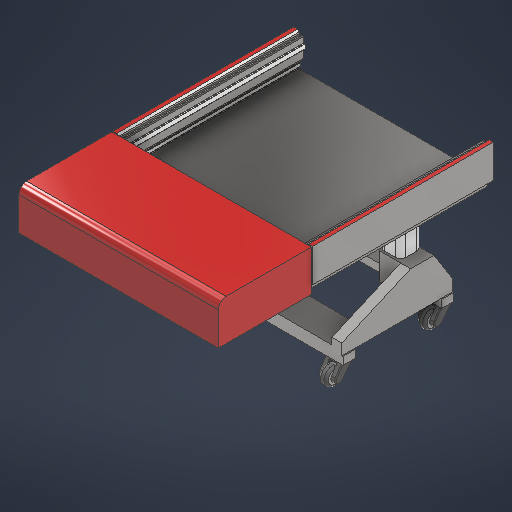
# Autodesk Inventor part: SACMI PH1500 POWER FEED SYSTEM
Saved by Autodesk Inventor 2025 (Build 290162000, 162)
## iProperties
Created: 2024-05-03
Part Number: SACMI PH1500 POWER FEED SYSTEM
Material: Generic
Document SubType Name: Modeling
Designer: zulet
Density: 1 g/cm^3
Appearance: Steel - Polished
Author: zulet
Autodesk Inventor part; units mm, degrees
ref_plane "YZ Plane" through (0, 0, 0) normal (1, 0, 0) x (0, 1, 0)
ref_plane "XZ Plane" through (0, 0, 0) normal (0, 1, 0) x (-1, 0, 0)
ref_plane "XY Plane" through (0, 0, 0) normal (0, 0, 1) x (1, 0, 0)
sketch "Sketch1" plane through (0, 0, 0) normal (0, 1, 0) x (-1, 0, 0)
  line L0 (700, -390) -> (-700, -390)
  line L1 (-700, -390) -> (-700, -500)
  line L2 (-700, -500) -> (700, -500)
  line L3 (700, -500) -> (700, -390)
  line L4 (0, 0) -> (0, -500) construction
  line L5 (0, 0) -> (-700, 0) construction
  line L6 (700, 390) -> (-700, 390)
  line L7 (-700, 390) -> (-700, 500)
  line L8 (-700, 500) -> (700, 500)
  line L9 (700, 500) -> (700, 390)
  point P0 (0, 500)
  dimension "d0" = 1400
  dimension "d1" = 500
  dimension "d2" = 110
  constraints: 20 end point, 5 symmetric about line, 2 horizontal, 2 parallel, 1 midpoint, 1 perpendicular, 1 point on line, 1 vertical
  measures "d0" distance of L1.end L2.end
  measures "d1" distance of L4.start L4.end
  measures "d2" distance between parallel lines of L0 L2
extrude "Extrusion1" add sketch "Sketch1" along normal blind 70
sketch "Sketch2" plane through (700, 0, 500) normal (1, 0, 0) x (0, 0, -1)
  line L0 (-1602.6406, 1986.5614) -> (1424.7743, 1986.5614) construction
  line L1 (1424.7743, 1986.5614) -> (1424.7743, -298.4008) construction
  line L2 (1424.7743, -298.4008) -> (-1602.6406, -298.4008) construction
  line L3 (-1602.6406, -298.4008) -> (-1602.6406, 1986.5614) construction
  line L4 (1917.7715, 602.0909) -> (1917.7715, -167.9091) construction
  line L5 (890, 70) -> (1000, 70) projected
  line L6 (0, 0) -> (0, 70) projected
  line L7 (1000, 70) -> (0, 70)
  line L8 (0, 70) -> (0, 170)
  line L9 (0, 170) -> (620, 440)
  line L10 (620, 440) -> (830, 440)
  line L11 (830, 440) -> (1000, 170)
  line L12 (1000, 170) -> (1000, 70)
  point P0 (500, 0)
  dimension "d10" = 770
  dimension "d30" = 2284.9623
  dimension "d45" = 100
  dimension "d46" = 210
  dimension "d47" = 270
  dimension "d48" = 620
  dimension "d49" = 100
  constraints: 14 end point, 2 parallel, 2 perpendicular, 1 horizontal, 1 vertical, 2 other
  measures "d10" distance of L4.start L4.end
  measures "d30" distance of L0.end L1.end
  measures "d45" distance of L6.end L8.end
  measures "d46" distance of L9.end L10.end
  measures "d47" vertical distance of L8.end L9.end
  measures "d48" horizontal distance of L8.end L9.end
  measures "d49" distance of L11.end L5.end
extrude "Extrusion2" add sketch "Sketch2" against normal blind 90
sketch "Sketch5" plane through (610, 0, 500) normal (-1, 0, 0) x (0, 0, 1)
  line L0 (-830, 440) -> (-1000, 170) projected
  line L1 (-830, 440) -> (-620, 440)
  line L2 (-620, 440) -> (-620, 200)
  line L3 (-620, 200) -> (-830, 200)
  line L4 (-830, 200) -> (-830, 440)
  point P0 (-500, 0)
  dimension "d57" = 210
  dimension "d58" = 240
  constraints: 8 end point, 2 parallel, 1 horizontal, 1 perpendicular
  measures "d57" distance of L2.end L3.end
  measures "d58" distance of L1.end L2.end
extrude "Extrusion5" add sketch "Sketch5" along normal blind 210
sketch "Sketch6" plane through (700, 440, -120) normal (0, 1, 0) x (1, 0, 0)
  line L0 (0, 0) -> (-90, 0) construction
  line L1 (-300, 0) -> (-300, 210) construction
  line L2 (-90, 0) -> (-300, 210) construction
  line L3 (-90, 210) -> (-90, 380) construction
  line L4 (-300, 0) -> (-90, 210) construction
  circle A0 centre (-195, 105) radius 65
  point P0 (-700, -120)
  dimension "d61" = 130
  constraints: 4 end point, 1 centre point, 1 midpoint
  measures "d61" diameter of A0
extrude "Extrusion6" add sketch "Sketch6" along normal blind 10
sketch "Sketch7" plane through (505, 450, -225) normal (0, 1, 0) x (1, 0, 0)
  line L0 (-95, -95) -> (95, -95)
  line L1 (95, -95) -> (95, 95)
  line L2 (95, 95) -> (-95, 95)
  line L3 (-95, 95) -> (-95, -95)
  circle A0 centre (0, 0) radius 65 projected
  line L4 (-95, -95) -> (95, 95) construction
  line L5 (95, -95) -> (-95, 95) construction
  point P0 (-505, -225)
  dimension "d64" = 190
  dimension "d65" = 190
  constraints: 12 end point, 2 midpoint, 2 parallel, 1 horizontal, 1 perpendicular
  measures "d64" distance of L2.end L1.end
  measures "d65" distance of L1.end L0.end
extrude "Extrusion7" add sketch "Sketch7" along normal blind 230 contours L3 L2 L1 L0 | A0
sketch "Sketch8" plane through (505, 680, -225) normal (0, 1, 0) x (1, 0, 0)
  circle A0 centre (0, 0) radius 65 projected
  point P0 (-505, -225)
extrude "Extrusion8" add sketch "Sketch8" along normal blind 207
fillet "Fillet1" radius 45 4 edges at (410, 565, -130) (410, 565, -320) (600, 565, -130) (600, 565, -320)
fillet "Fillet2" radius 20 2 edges at (400, 320, -330) (400, 320, -120)
mirror "Mirror1" about plane through (0, 0, 0) normal (1, 0, 0) of "Extrusion2", "Extrusion5", "Extrusion6", "Extrusion7", "Extrusion8", "Fillet1", "Fillet2"
sketch "Sketch9" plane through (505, 887, -225) normal (0, 1, 0) x (1, 0, 0)
  line L0 (345, 440) -> (-1355, 440)
  line L1 (-1355, 440) -> (-1355, -1190)
  line L2 (-1355, -1190) -> (345, -1190)
  line L3 (345, -1190) -> (345, 440)
  line L4 (345, 440) -> (-1355, -1190) construction
  line L5 (-1355, 440) -> (345, -1190) construction
  line L6 (-505, -225) -> (-505, -375) construction
  dimension "d72" = 1630
  dimension "d73" = 1700
  dimension "d74" = 150
  constraints: 14 end point, 2 midpoint, 2 parallel, 1 horizontal, 1 perpendicular, 1 vertical
  measures "d72" distance of L0.end L1.end
  measures "d73" distance of L0.start L0.end
  measures "d74" distance of L6.start L6.end
extrude "Extrusion9" add sketch "Sketch9" along normal blind 70
sketch "Sketch10" plane through (505, 957, -225) normal (0, 1, 0) x (1, 0, 0)
  line L0 (-2534.8572, 1233.6299) -> (1500.9888, 1233.6299) construction
  line L1 (1500.9888, 1233.6299) -> (1500.9888, -2836.0091) construction
  line L2 (1500.9888, -2836.0091) -> (-2534.8572, -2836.0091) construction
  line L3 (-2534.8572, -2836.0091) -> (-2534.8572, 1233.6299) construction
  line L4 (-4550.9548, -1760.3211) -> (-2210.9548, -1760.3211)
  line L5 (-1355, -1190) -> (345, -1190) projected
  line L6 (345, -1190) -> (395, -1190)
  line L7 (395, -1190) -> (395, 440)
  line L8 (395, 440) -> (345, 440)
  line L9 (345, 440) -> (345, -1190)
  point P0 (-505, -225)
  dimension "d88" = 2340
  dimension "d113" = 4035.8459
  dimension "d125" = 50
  dimension "d126" = 1630
  constraints: 10 end point, 3 horizontal, 2 parallel, 1 perpendicular, 2 other
  measures "d88" distance of L4.start L4.end
  measures "d113" distance of L1.end L2.end
  measures "d125" distance of L8.end L7.end
  measures "d126" distance of L7.end L6.end
extrude "Extrusion10" add sketch "Sketch10" along normal blind 300 and the other way blind 50
chamfer "Chamfer1" distance 50 angle 45 1 edges at (900, 907, 150)
sketch "Sketch12" plane through (-700, 0, -500) normal (-1, 0, 0) x (0, 0, 1)
  line L0 (890, 0) -> (1000, 0) projected
  line L1 (890, 0) -> (994.4657, -126.554)
  line L2 (1000, 0) -> (1053.9917, -82.7883)
  arc A0 (994.4657, -126.554) -> (1053.9917, -82.7883) centre (1023, -103) ccw
  point P0 (500, 0)
  dimension "d134" = 103
  dimension "d135" = 23
  dimension "d136" = 37
  constraints: 4 end point, 2 point on circle, 2 tangent, 1 centre point
  measures "d134" distance from line of L0 A0.centre
  measures "d135" horizontal distance of L0.end A0.centre
  measures "d136" radius of A0
extrude "Extrusion11" add sketch "Sketch12" against normal blind 40
sketch "Sketch13" plane through (-660, 0, -500) normal (1, 0, 0) x (0, 0, -1)
  arc A0 (-1053.9917, -82.7883) -> (-994.4657, -126.554) centre (-1023, -103) ccw projected
  circle A1 centre (-1023, -103) radius 80
  point P0 (-500, 0)
  dimension "d139" = 160
  constraints: 1 centre point, 1 coincident
  measures "d139" diameter of A1
extrude "Extrusion12" add sketch "Sketch13" along normal blind 70
sketch "Sketch14" plane through (-590, -103, 523) normal (1, 0, 0) x (0, 0, -1)
  line L0 (133, 103) -> (28.5343, -23.554) projected
  arc A0 (-30.9917, 20.2117) -> (28.5343, -23.554) centre (0, 0) ccw projected
  line L1 (-30.9917, 20.2117) -> (23, 103) projected
  line L2 (23, 103) -> (133, 103) projected
  line L3 (11.9132, 86) -> (118.9671, 86)
  point P0 (523, 103)
  dimension "d142" = 17
  constraints: 2 end point, 2 point on line, 1 parallel
  measures "d142" distance between parallel lines of L2 L3
extrude "Extrusion13" add sketch "Sketch14" along normal blind 40
extrude "Extrusion14" add sketch "Sketch14" against normal blind 70 contours L0 L3 L1 L2
sketch "Sketch15" plane through (-700, 0, -500) normal (-1, 0, 0) x (0, 0, 1)
  line L0 (994.4657, -126.554) -> (890, 0) projected
  line L1 (1053.9917, -82.7883) -> (1000, 0) projected
  line L2 (890, 0) -> (1000, 0)
  line L3 (1000, 70) -> (890, 70) projected
  line L4 (890, 70) -> (1000, 70)
  line L5 (890, 0) -> (890, 70) projected
  line L6 (1000, 0) -> (1000, 170) projected
  point P0 (500, 0)
  constraints: 4 end point, 1 collinear, 1 horizontal
extrude "Extrusion15" add sketch "Sketch15" along normal blind 10
fillet "Fillet3" radius 20 4 edges at (-660, -156.757, 582.2468) (-660, -87.1101, 444.5939) (-590, -156.757, 582.2468) (-590, -87.1101, 444.5939)
fillet "Fillet4" radius 7 8 edges at (-700, -132.8099, 544.9174) (-700, -63.277, 442.2328) (-700, -41.3941, 526.9959) (-550, -132.8099, 544.9174) (-550, -63.277, 442.2328) (-550, -41.3941, 526.9959) (-625, -17, 511.0868) (-625, -17, 404.0329)
mirror "Mirror2" about plane through (0, 0, 0) normal (1, 0, 0) of "Extrusion11", "Extrusion12", "Extrusion13", "Extrusion14", "Extrusion15", "Fillet3", "Fillet4"
pattern_linear "Rectangular Pattern1" count 2 spacing 890 along (0, 0, -1) of "Extrusion11", "Extrusion12", "Extrusion13", "Extrusion14", "Extrusion15", "Fillet3", "Fillet4", "Mirror2"
sketch "Sketch17" plane through (-850, 887, 965) normal (0, 0, 1) x (1, 0, 0)
  line L0 (1700, 70) -> (1700, 370) projected
  line L1 (1700, 90) -> (1690, 90)
  line L2 (1690, 90) -> (1690, 120)
  line L3 (1690, 120) -> (1700, 120)
  line L4 (1700, 120) -> (1700, 90)
  line L5 (0, 70) -> (1700, 70) projected
  circle A0 centre (1695, 120) radius 3
  circle A1 centre (1695, 90) radius 3
  line L6 (1700, 370) -> (1660, 370)
  line L7 (1660, 370) -> (1660, 170)
  line L8 (1660, 170) -> (1700, 170)
  line L9 (1700, 170) -> (1700, 370)
  line L10 (1660, 290) -> (1645, 290)
  line L11 (1645, 290) -> (1645, 250)
  line L12 (1645, 250) -> (1660, 250)
  line L13 (1660, 250) -> (1660, 290)
  circle A2 centre (1652.5, 250) radius 5
  circle A3 centre (1652.5, 290) radius 5
  line L14 (1660, 340) -> (1700, 340)
  line L15 (1675, 340) -> (1685, 340)
  line L16 (1685, 340) -> (1685, 330)
  line L17 (1685, 330) -> (1675, 330)
  line L18 (1675, 330) -> (1675, 340)
  point P0 (850, -887)
  point P1 (1692, 90)
  point P2 (1698, 90)
  point P3 (1698, 120)
  point P4 (1692, 120)
  point P5 (1660, 270)
  point P6 (1657.5, 290)
  point P7 (1647.5, 290)
  point P8 (1647.5, 250)
  point P9 (1657.5, 250)
  point P10 (1680, 340)
  dimension "d154" = 10
  dimension "d155" = 30
  dimension "d156" = 20
  dimension "d157" = 6
  dimension "d158" = 6
  dimension "d161" = 40
  dimension "d162" = 200
  dimension "d163" = 40
  dimension "d164" = 15
  dimension "d165" = 10
  dimension "d166" = 10
  dimension "d167" = 30
  dimension "d168" = 10
  dimension "d169" = 10
  constraints: 34 end point, 8 midpoint, 8 parallel, 5 horizontal, 4 centre point, 4 perpendicular, 4 point on line
  measures "d154" distance of L2.end L3.end
  measures "d155" distance of L1.end L2.end
  measures "d156" distance between parallel lines of L5 L1
  measures "d157" diameter of A0
  measures "d158" diameter of A1
  measures "d161" distance of L8.end L7.end
  measures "d162" distance of L7.end L6.end
  measures "d163" distance of L10.end L11.end
  measures "d164" distance of L11.end L12.end
  measures "d165" diameter of A2
  measures "d166" diameter of A3
  measures "d167" distance between parallel lines of L14 L6
  measures "d168" distance of L16.end L17.end
  measures "d169" distance of L15.end L16.end
extrude "Extrusion16" add sketch "Sketch17" against normal up to surface (1630 mm away) contours L1 A1 L2 L3 A0 L0 | L8 L7 L14 L18 L17 L16 L0 | L12 A2 L11 L10 A3 L7
sketch "Sketch18" plane through (-850, 887, 965) normal (0, 0, 1) x (1, 0, 0)
  line L0 (1670, 320) -> (1740, 320)
  line L1 (1740, 320) -> (1740, 180)
  line L2 (1740, 180) -> (1670, 180)
  line L3 (1670, 180) -> (1670, 320)
  line L4 (1660, 340) -> (1660, 290) projected
  line L5 (1660, 170) -> (1700, 170) projected
  line L6 (1750, 70) -> (1750, 370) projected
  line L7 (1685, 330) -> (1675, 330) projected
  point P0 (850, -887)
  point P1 (1680, 330)
  dimension "d170" = 10
  dimension "d171" = 10
  dimension "d172" = 10
  dimension "d173" = 10
  constraints: 8 end point, 2 parallel, 1 horizontal, 1 midpoint, 1 perpendicular
  measures "d170" distance between parallel lines of L4 L3
  measures "d171" distance between parallel lines of L5 L2
  measures "d172" distance between parallel lines of L6 L1
  measures "d173" distance from line of point (1680, 330) L0
extrude "Extrusion17" cut sketch "Sketch18" against normal through all
chamfer "Chamfer2" distance 15 angle 45 1 edges at (850, 1257, 150)
mirror "Mirror3" about plane through (0, 0, 0) normal (1, 0, 0) of "Extrusion10", "Chamfer1", "Extrusion16", "Extrusion17", "Chamfer2"
sketch "Sketch19" plane through (-850, 887, 965) normal (0, 0, 1) x (1, 0, 0)
  line L0 (-50, 370) -> (1750, 370)
  line L1 (1750, 370) -> (1750, 0)
  line L2 (1750, 0) -> (-50, 0)
  line L3 (-50, 0) -> (-50, 370)
  point P0 (850, -887)
  dimension "d179" = 1800
  dimension "d180" = 370
  constraints: 8 end point, 2 parallel, 1 horizontal, 1 perpendicular
  measures "d179" distance of L1.end L2.end
  measures "d180" distance of L0.end L1.end
extrude "Extrusion18" add sketch "Sketch19" along normal blind 850
fillet "Fillet5" radius 70 1 edges at (0, 1257, 1815)
fillet "Fillet6" radius 3 1 edges at (0, 957, -665)
sketch "Sketch20" plane through (0, 70, 0) normal (0, 1, 0) x (1, 0, 0)
  line L0 (610, 500) -> (-610, 500) projected
  line L1 (-610, -500) -> (610, -500) projected
  line L2 (557, -390) -> (-557, -390) projected
  line L3 (-610, -390) -> (-610, -500) projected
  line L4 (-610, -500) -> (610, -500) projected
  line L5 (610, -500) -> (610, -390) projected
  line L6 (610, -390) -> (-610, -390) projected
  line L7 (610, -500) -> (-610, -500)
  line L8 (-610, -500) -> (-610, -220)
  line L9 (-610, -220) -> (610, -220)
  line L10 (610, -220) -> (610, -500)
  line L11 (610, -500) -> (610, -390) projected
  point P0 (0, 0)
  dimension "d186" = 170
  constraints: 8 end point, 2 collinear, 2 parallel, 1 horizontal, 1 perpendicular, 1 point on line
  measures "d186" distance between parallel lines of L2 L9
extrude "Extrusion19" add sketch "Sketch20" along normal blind 40
sketch "Sketch21" plane through (0, 110, 0) normal (0, 1, 0) x (1, 0, 0)
  line L0 (0, 0) -> (0, -500) construction
  line L1 (-610, -500) -> (610, -500) construction
  circle A0 centre (0, -270) radius 37.5
  circle A1 centre (0, -410) radius 55
  line L2 (610, -220) -> (-610, -220) projected
  dimension "d189" = 75
  dimension "d190" = 110
  dimension "d191" = 50
  dimension "d192" = 90
  constraints: 2 centre point, 2 end point, 2 point on line, 1 midpoint
  measures "d189" diameter of A0
  measures "d190" diameter of A1
  measures "d191" distance from line of L2 A0.centre
  measures "d192" distance from line of L1 A1.centre
extrude "Extrusion20" add sketch "Sketch21" along normal blind 240
sketch "Sketch22" plane through (0, 350, 410) normal (0, 1, 0) x (1, 0, 0)
  circle A0 centre (0, 140) radius 37.5 construction
  line L0 (0, 177.5) -> (0, -55) construction
  circle A1 centre (0, 0) radius 55 construction
  line L1 (250, 311.25) -> (-250, 311.25)
  line L2 (-250, 311.25) -> (-250, -188.75)
  line L3 (-250, -188.75) -> (250, -188.75)
  line L4 (250, -188.75) -> (250, 311.25)
  line L5 (250, 311.25) -> (-250, -188.75) construction
  line L6 (-250, 311.25) -> (250, -188.75) construction
  point P0 (0, 410)
  point P1 (0, 61.25)
  dimension "d195" = 500
  dimension "d196" = 500
  constraints: 14 end point, 3 midpoint, 2 parallel, 2 point on line, 2 vertical alignment, 1 horizontal, 1 perpendicular, 2 other
  measures "d195" distance of L3.end L2.end
  measures "d196" distance of L2.end L1.end
extrude "Extrusion21" add sketch "Sketch22" along normal blind 414
sketch "Sketch23" plane through (-250, 350, 598.75) normal (0, 0, 1) x (1, 0, 0)
  line L0 (0, 414) -> (500, 414) construction
  line L1 (250, 414) -> (250, 0) construction
  line L2 (500, 0) -> (0, 0) construction
  line L3 (110, 94) -> (390, 94)
  line L4 (390, 94) -> (390, 414)
  line L5 (390, 414) -> (110, 414)
  line L6 (110, 414) -> (110, 94)
  line L7 (110, 94) -> (390, 414) construction
  line L8 (390, 94) -> (110, 414) construction
  point P0 (250, -350)
  point P1 (250, 254)
  dimension "d199" = 280
  dimension "d200" = 320
  constraints: 14 end point, 4 midpoint, 2 parallel, 2 point on line, 1 horizontal, 1 perpendicular
  measures "d199" distance of L3.start L3.end
  measures "d200" distance of L3.end L4.end
extrude "Extrusion22" add sketch "Sketch23" along normal blind 415
sketch "Sketch24" plane through (0, 764, 410) normal (0, 1, 0) x (1, 0, 0)
  line L0 (140, -603.75) -> (-140, -603.75) construction
  line L1 (0, -603.75) -> (0, 311.25) construction
  line L2 (250, 311.25) -> (-250, 311.25) construction
  circle A0 centre (0, -338.75) radius 75
  line L3 (-250, -188.75) -> (-140, -188.75) construction
  point P0 (0, 410)
  dimension "d203" = 150
  dimension "d204" = 150
  constraints: 2 end point, 2 midpoint, 1 centre point, 1 point on line
  measures "d203" diameter of A0
  measures "d204" distance from line of L3 A0.centre
extrude "Extrusion23" add sketch "Sketch24" along normal up to surface (123 mm away)
fillet "Fillet7" radius 50 6 edges at (-250, 557, 98.75) (-250, 557, 598.75) (250, 557, 598.75) (250, 557, 98.75) (-140, 604, 1013.75) (140, 604, 1013.75)
fillet "Fillet8" radius 30 6 edges at (-37.5, 350, 270) (-55, 350, 410) (-75, 887, 748.75) (-140, 604, 598.75) (0, 444, 598.75) (140, 604, 598.75)
sketch "Sketch25" plane through (0, 764, 410) normal (0, 1, 0) x (1, 0, 0)
  arc A0 (90, -603.75) -> (140, -553.75) centre (90, -553.75) ccw projected
  line L0 (140, -218.75) -> (140, -553.75) projected
  arc A1 (170, -188.75) -> (140, -218.75) centre (170, -218.75) ccw projected
  line L1 (170, -188.75) -> (200, -188.75) projected
  arc A2 (200, -188.75) -> (250, -138.75) centre (200, -138.75) ccw projected
  line L2 (250, -138.75) -> (250, 261.25) projected
  arc A3 (250, 261.25) -> (200, 311.25) centre (200, 261.25) ccw projected
  line L3 (200, 311.25) -> (-200, 311.25) projected
  arc A4 (-200, 311.25) -> (-250, 261.25) centre (-200, 261.25) ccw projected
  line L4 (-250, 261.25) -> (-250, -138.75) projected
  arc A5 (-250, -138.75) -> (-200, -188.75) centre (-200, -138.75) ccw projected
  line L5 (-200, -188.75) -> (-170, -188.75) projected
  arc A6 (-140, -218.75) -> (-170, -188.75) centre (-170, -218.75) ccw projected
  line L6 (-140, -218.75) -> (-140, -553.75) projected
  arc A7 (-140, -553.75) -> (-90, -603.75) centre (-90, -553.75) ccw projected
  line L7 (90, -603.75) -> (-90, -603.75) projected
  circle A8 centre (0, -338.75) radius 75 projected
  line L8 (230, 261.25) -> (230, -138.75)
  arc A9 (200, -168.75) -> (230, -138.75) centre (200, -138.75) ccw
  line L9 (200, -168.75) -> (170, -168.75)
  arc A10 (170, -168.75) -> (120, -218.75) centre (170, -218.75) ccw
  line L10 (120, -218.75) -> (120, -553.75)
  arc A11 (90, -583.75) -> (120, -553.75) centre (90, -553.75) ccw
  line L11 (90, -583.75) -> (-90, -583.75)
  arc A12 (-120, -553.75) -> (-90, -583.75) centre (-90, -553.75) ccw
  line L12 (-120, -553.75) -> (-120, -218.75)
  arc A13 (-120, -218.75) -> (-170, -168.75) centre (-170, -218.75) ccw
  line L13 (-170, -168.75) -> (-200, -168.75)
  arc A14 (-230, -138.75) -> (-200, -168.75) centre (-200, -138.75) ccw
  line L14 (-230, -138.75) -> (-230, 261.25)
  arc A15 (-200, 291.25) -> (-230, 261.25) centre (-200, 261.25) ccw
  line L15 (-200, 291.25) -> (200, 291.25)
  arc A16 (230, 261.25) -> (200, 291.25) centre (200, 261.25) ccw
  line L16 (170, -168.75) -> (-170, -168.75)
  point P0 (0, 410)
  dimension "d209" = 20
  constraints: 18 end point, 16 point on circle, 8 centre point, 1 point on line, 15 other
  measures "d209" distance between parallel lines of L2 L8
extrude "Extrusion24" cut sketch "Sketch25" against normal blind 390 contours L8 A9 L9 L16 L13 A14 L14 A15 L15 A16
sketch "Sketch26" plane through (-900, 957, -665) normal (-1, 0, 0) x (0, 0, 1)
  line L0 (2410, 300) -> (0, 300) projected
  line L1 (1630, -70) -> (1640, -70)
  line L2 (1640, -70) -> (1640, 300)
  line L3 (1640, 300) -> (1630, 300)
  line L4 (1630, 300) -> (1630, -70)
  point P0 (665, -957)
  dimension "d212" = 10
  constraints: 8 end point, 2 parallel, 1 horizontal, 1 perpendicular, 1 point on line
  measures "d212" distance between parallel lines of L2 L4
extrude "Extrusion25" cut sketch "Sketch26" against normal blind 10
sketch "Sketch27" plane through (505, 1257, -225) normal (0, 1, 0) x (1, 0, 0)
  line L0 (-1405, -1190) -> (-1395, -1190) projected
  line L1 (-1405, -1190) -> (395, -1190)
  line L2 (395, -1190) -> (395, -1200)
  line L3 (395, -1200) -> (-1405, -1200)
  line L4 (-1405, -1200) -> (-1405, -1190)
  line L5 (395, 440) -> (395, -1970) projected
  point P0 (-505, -225)
  dimension "d215" = 10
  constraints: 8 end point, 2 parallel, 1 collinear, 1 horizontal, 1 perpendicular
  measures "d215" distance between parallel lines of L3 L1
extrude "Extrusion26" cut sketch "Sketch27" against normal blind 10
sketch "Sketch28" plane through (505, 887, -225) normal (0, -1, 0) x (1, 0, 0)
  line L0 (-1395, 1200) -> (-1395, 1190) projected
  line L1 (395, 1200) -> (-1395, 1200) projected
  line L2 (395, 1190) -> (395, 1200) projected
  line L3 (350, 1190) -> (395, 1190) projected
  line L4 (-1360, 1190) -> (350, 1190) projected
  line L5 (-1395, 1190) -> (-1360, 1190) projected
  point P0 (-505, 225)
extrude "Extrusion27" cut sketch "Sketch28" against normal blind 10
sketch "Sketch29" plane through (900, 957, -665) normal (1, 0, 0) x (0, 0, -1)
  line L0 (-1630, -60) -> (-1640, -60) projected
  line L1 (-1640, 290) -> (-1640, -60) projected
  line L2 (-1640, 290) -> (-1630, 290) projected
  line L3 (-1630, 250) -> (-1630, 290) projected
  line L4 (-1630, 110) -> (-1630, 250) projected
  line L5 (-1630, -10) -> (-1630, 110) projected
  line L6 (-1630, -60) -> (-1630, -10) projected
  point P0 (-665, -957)
extrude "Extrusion28" cut sketch "Sketch29" against normal blind 10
equation "\"d49\" = d45"
body "Solid1"
